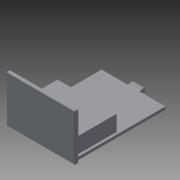
# Autodesk Inventor part: BOTTOM
Saved by Autodesk Inventor 2014 SP1 (Build 180222100, 222)
## iProperties
Created: 2013-12-02
Part Number: BOTTOM
Material: Generic
Document SubType Name: Modeling
Designer: Dominik
Density: 1 g/cm^3
Appearance: Default
Author: Dominik
Autodesk Inventor part; units mm, degrees
ref_plane "YZ Plane" through (0, 0, 0) normal (1, 0, 0) x (0, 1, 0)
ref_plane "XZ Plane" through (0, 0, 0) normal (0, 1, 0) x (-1, 0, 0)
ref_plane "XY Plane" through (0, 0, 0) normal (0, 0, 1) x (1, 0, 0)
sketch "Sketch1" plane through (0, 0, 0) normal (0, 0, 1) x (1, 0, 0)
  line L0 (0, 0) -> (55, 0)
  line L1 (55, 0) -> (55, 80)
  line L2 (55, 80) -> (0, 80)
  line L3 (0, 80) -> (0, 0)
  dimension "d0" = 55
  dimension "d1" = 80
  constraints: 8 end point
  measures "d0" distance between parallel lines of L1 L3
  measures "d1" distance between parallel lines of L0 L2
extrude "Extrusion1" add sketch "Sketch1" along normal blind 3
sketch "Sketch2" plane through (0, 0, 3) normal (0, 0, 1) x (1, 0, 0)
  line L0 (55, 0) -> (55, 80) projected
  line L1 (0, 80) -> (0, 0) projected
  line L2 (-2, 0) -> (57, 0)
  line L3 (57, 0) -> (57, 3)
  line L4 (57, 3) -> (-2, 3)
  line L5 (-2, 3) -> (-2, 0)
  dimension "d4" = 3
  dimension "d5" = 2
  dimension "d6" = 2
  constraints: 8 end point
  measures "d4" distance between parallel lines of L2 L4
  measures "d5" distance between parallel lines of L3 L0
  measures "d6" distance between parallel lines of L5 L1
extrude "Extrusion2" add sketch "Sketch2" along normal blind 37.5 and the other way blind 3
sketch "Sketch4" plane through (0, 80, 0) normal (0, 1, 0) x (1, 0, 0)
  line L0 (55, -3) -> (0, -3) projected
  line L1 (55, 0) -> (55, -3) projected
  line L2 (0, 0) -> (22.5, 0) construction
  line L3 (22.5, 0) -> (22.5, -3) construction
  line L4 (22.5, -3) -> (0, -3) construction
  line L5 (0, -3) -> (0, 0) construction
  line L6 (55, 0) -> (32.5, 0) construction
  line L7 (32.5, 0) -> (32.5, -3) construction
  line L8 (32.5, -3) -> (55, -3) construction
  line L9 (55, -3) -> (55, 0) construction
  line L10 (22.5, 0) -> (32.5, 0)
  line L11 (32.5, 0) -> (32.5, -3)
  line L12 (32.5, -3) -> (22.5, -3)
  line L13 (22.5, -3) -> (22.5, 0)
  dimension "d15" = 22.5
  dimension "d16" = 22.5
  dimension "d17" = 10
  constraints: 24 end point, 2 point on line
  measures "d15" distance between parallel lines of L3 L5
  measures "d16" distance between parallel lines of L1 L7
  measures "d17" distance between parallel lines of L7 L3
extrude "Extrusion4" add sketch "Sketch4" along normal blind 5
sketch "Sketch5" plane through (0, 0, 3) normal (0, 0, 1) x (1, 0, 0)
  line L0 (32.5, 80) -> (32.5, 85) projected
  line L1 (22.5, 85) -> (32.5, 85)
  line L2 (32.5, 85) -> (32.5, 82.1)
  line L3 (32.5, 82.1) -> (22.5, 82.1)
  line L4 (22.5, 82.1) -> (22.5, 85)
  point P0 (0, 0)
  dimension "d20" = 2.9
  constraints: 8 end point, 1 point on line
  measures "d20" distance between parallel lines of L3 L1
extrude "Extrusion5" add sketch "Sketch5" along normal blind 1
chamfer "Chamfer1" distance 1 distance2 1 1 edges at (27.5, 82.1, 4) measured on face at (27.5, 82.6, 4)
chamfer "Chamfer2" distance 1.9 distance2 1 1 edges at (27.5, 85, 4) measured on face at (27.5, 84.5, 4)
sketch "Sketch6" plane through (0, 0, 3) normal (0, 0, 1) x (1, 0, 0)
  line L0 (0, 80) -> (0, 3) projected
  line L1 (0, 3) -> (55, 3) projected
  line L2 (55, 3) -> (55, 80) projected
  line L3 (2, 3) -> (53, 3)
  line L4 (53, 3) -> (53, 40)
  line L5 (53, 40) -> (2, 40)
  line L6 (2, 40) -> (2, 3)
  point P0 (0, 0)
  dimension "d29" = 37
  dimension "d30" = 2
  dimension "d31" = 2
  constraints: 8 end point, 2 vertical, 1 horizontal, 1 point on line
  measures "d29" distance between parallel lines of L1 L5
  measures "d30" distance between parallel lines of L2 L4
  measures "d31" distance between parallel lines of L0 L6
extrude "Extrusion6" add sketch "Sketch6" along normal blind 13.5
fillet "Fillet1" radius 1 4 edges at (32.5, 83.1, 4) (22.5, 83.1, 4) (27.5, 83.1, 4) (27.5, 83.0999, 4)
chamfer "Chamfer3" distance 0.5 angle 45 12 edges at (0, 41.5, 0) (11.25, 80, 0) (22.5, 82.5, 0) (27.5, 85, 0) (32.5, 82.5, 0) (43.75, 80, 0) (55, 41.5, 0) (-1, 3, 0) (-2, 1.5, 0) (27.5, 0, 0) (57, 1.5, 0) (56, 3, 0)
chamfer "Chamfer4" distance 0.5 angle 45 3 edges at (-2, 0, 20.5) (27.5, 0, 40.5) (57, 0, 20.5)
chamfer "Chamfer5" distance 0.5 angle 45 3 edges at (-2, 1.75, 40.5) (27.5, 3, 40.5) (57, 1.75, 40.5)
equation "\"d16\" = d15"
equation "\"d31\" = d30"
body "Solid1"
